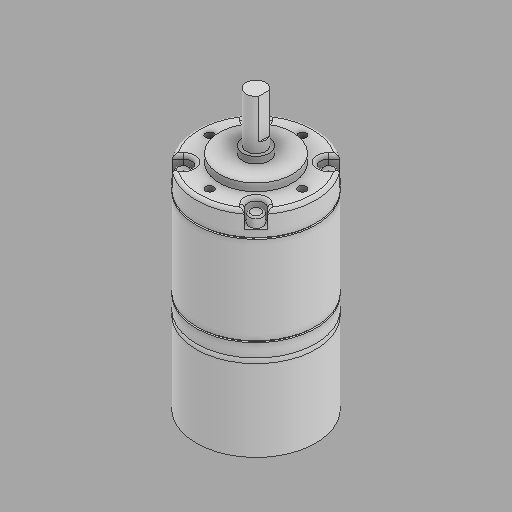
# Autodesk Inventor part: BLDC_3626
Saved by Autodesk Inventor 2025 (Build 290162000, 162)
## iProperties
Created: 2025-04-08
Part Number: BLDC_3626
Material: Типовые
Document SubType Name: Modeling
Designer: Artem Sannikov
Density: 1 g/cm^3
Appearance: По умолчанию
Author: Artem Sannikov
Autodesk Inventor part; units mm, degrees
ref_plane "YZ Plane" through (0, 0, 0) normal (1, 0, 0) x (0, 1, 0)
ref_plane "XZ Plane" through (0, 0, 0) normal (0, 1, 0) x (-1, 0, 0)
ref_plane "XY Plane" through (0, 0, 0) normal (0, 0, 1) x (1, 0, 0)
sketch "Эскиз1" plane through (0, 0, 0) normal (1, 0, 0) x (0, 1, 0)
  line L0 (0, 0) -> (734.8739, 0) construction
  line L1 (0, 0) -> (26, 0)
  line L2 (26, 0) -> (26, -16.5)
  line L3 (24.5, -18) -> (0, -18)
  line L4 (0, -18) -> (0, -6.5)
  arc A0 (24.5, -18) -> (26, -16.5) centre (24.5, -16.5) ccw
  line L5 (0, 0) -> (-3, 0)
  line L6 (-3, 0) -> (-3, -6.5)
  line L7 (-3, -6.5) -> (0, -6.5)
  line L8 (6.8488, -18) -> (80.5984, -18) construction
  line L9 (26, 0) -> (64.5, 0)
  line L10 (64.5, -11) -> (64.5, -18)
  line L11 (26, -18) -> (26, 0)
  line L12 (30.5, -18) -> (30.5, -17.5)
  line L13 (30.5, -17.5) -> (30, -17.5)
  line L14 (30, -17.5) -> (30, -18)
  line L15 (57, -18) -> (57, -17.5)
  line L16 (57, -17.5) -> (57.5, -17.5)
  line L17 (57.5, -17.5) -> (57.5, -18)
  line L18 (64.5, 0) -> (66.8, 0)
  line L19 (66.8, 0) -> (66.8, -11)
  line L20 (66.8, -11) -> (64.5, -11)
  line L21 (64.5, -18) -> (57.5, -18)
  line L22 (57, -18) -> (30.5, -18)
  line L23 (30, -18) -> (26, -18)
  line L24 (66.8, 0) -> (83.8, 0)
  line L25 (83.8, 0) -> (83.8, -3)
  line L26 (83.8, -3) -> (68.8, -3)
  line L27 (66.8, -3) -> (66.8, 0)
  line L28 (66.8, 0) -> (68.8, 0)
  line L29 (68.8, -3) -> (68.8, -4)
  line L30 (68.8, -4) -> (66.8, -4)
  line L31 (66.8, -4) -> (66.8, 0)
  line L32 (-3, -1.55) -> (-3.9167, -1.55)
  line L33 (-3.9167, -1.55) -> (-3.9167, 0)
  line L34 (-3.9167, 0) -> (-3, 0)
  point P0 (26, -18)
  point P1 (30, -17.75)
  point P2 (30.5, -17.75)
  dimension "d0" = 26
  dimension "d1" = 18
  dimension "d2" = 1.5
  dimension "d4" = 6.5
  dimension "d5" = 3
  dimension "d6" = 38.5
  dimension "d7" = 4
  dimension "d8" = 0.5
  dimension "d14" = 11
  dimension "d15" = 2.3
  dimension "d16" = 0.5
  dimension "d17" = 0.5
  dimension "d18" = 7
  dimension "d19" = 0.5
  dimension "d20" = 17
  dimension "d21" = 3
  dimension "d22" = 2
  dimension "d23" = 4
  dimension "d28" = 1.55
  constraints: 70 end point, 14 parallel, 8 horizontal, 8 perpendicular, 6 point on line, 2 midpoint, 2 point on circle, 2 tangent, 1 centre point
  measures "d0" distance of point (26, -18) L3.end
  measures "d1" distance of L1.end point (26, -18)
  measures "d2" radius of A0
  measures "d4" distance of L5.end L6.end
  measures "d5" distance between parallel lines of L4 L6
  measures "d6" distance of L10.end L11.start
  measures "d7" distance from line of point (30, -17.75) L11
  measures "d8" distance of point (30.5, -17.75) point (30, -17.75)
  measures "d14" distance of L18.end L19.end
  measures "d15" distance between parallel lines of L19 L10
  measures "d16" distance of L15.end L16.end
  measures "d17" distance of L16.end L17.end
  measures "d18" distance between parallel lines of L10 L17
  measures "d19" distance between parallel lines of L8 L13
  measures "d20" distance of L25.end L27.start
  measures "d21" distance between parallel lines of L0 L26
  measures "d22" distance of L29.end L30.end
  measures "d23" distance of L28.end L29.end
  measures "d28" distance between parallel lines of L32 L34
revolve "Вращение1" add sketch "Эскиз1" angle 360 about axis through (0, 0, 0) along (0, 1, 0)
sketch "Эскиз2" plane through (0, 83.8, 0) normal (0, 1, 0) x (1, 0, 0)
  circle A0 centre (0, 0) radius 3 projected
  line L0 (2.5, -1.6583) -> (5.0866, -1.6583)
  line L1 (5.0866, -1.6583) -> (5.0866, 2.9667)
  line L2 (5.0866, 2.9667) -> (2.5, 2.9667)
  line L3 (2.5, 2.9667) -> (2.5, -1.6583)
  point P0 (2.5, 1.6583)
  dimension "d25" = 5.5
  constraints: 8 end point, 2 parallel, 1 horizontal, 1 perpendicular, 2 other
extrude "Выдавливание1" cut sketch "Эскиз2" against normal blind 12 contours L3 A0 picked at (2.5914, 0.3806)
sketch "Эскиз3" plane through (0, 64.5, 0) normal (0, 1, 0) x (1, 0, 0)
  circle A0 centre (0, 0) radius 14 construction
  point P0 (0, 14)
  point P1 (-14, 0)
  point P2 (0, -14)
  point P3 (14, 0)
  dimension "d29" = 28
  dimension "d32" = 360
  constraints: 1 coincident, 1 vertical alignment, 7 other
hole "Отверстие1" at (0, 64.5, -14) at (-14, 64.5, 0) at (0, 64.5, 14) at (14, 64.5, 0) direction (0, -1, 0) diameter 2.459 depth 8.8 tip angle 118 thread size "M3x0.5" class "6H" standard "ISO Metric profile"
sketch "Эскиз4" plane through (0, 64.5, 0) normal (0, 1, 0) x (1, 0, 0)
  line L0 (0, 0) -> (18, 0) construction
  circle A0 centre (0, 0) radius 18 projected
  line L1 (0, 0) -> (12.7279, 12.7279) construction
  circle A1 centre (10.9602, 10.9602) radius 2.5
  line L2 (12.7279, 9.1924) -> (14.3723, 10.8368)
  line L3 (9.1924, 12.7279) -> (10.8368, 14.3723)
  line L4 (10.8368, 14.3723) -> (14.3723, 14.3723)
  line L5 (14.3723, 14.3723) -> (14.3723, 10.8368)
  line L6 (14.3723, 10.8368) -> (10.8368, 10.8368)
  line L7 (10.8368, 10.8368) -> (10.8368, 14.3723)
  line L8 (-9.1924, 12.7279) -> (-10.8368, 14.3723)
  circle A2 centre (-10.9602, 10.9602) radius 2.5
  line L9 (-10.8368, 14.3723) -> (-10.8368, 10.8368)
  line L10 (-10.8368, 10.8368) -> (-14.3723, 10.8368)
  line L11 (-12.7279, 9.1924) -> (-14.3723, 10.8368)
  line L12 (-14.3723, 10.8368) -> (-14.3723, 14.3723)
  line L13 (-14.3723, 14.3723) -> (-10.8368, 14.3723)
  line L14 (-12.7279, -9.1924) -> (-14.3723, -10.8368)
  circle A3 centre (-10.9602, -10.9602) radius 2.5
  line L15 (-14.3723, -10.8368) -> (-10.8368, -10.8368)
  line L16 (-10.8368, -10.8368) -> (-10.8368, -14.3723)
  line L17 (-9.1924, -12.7279) -> (-10.8368, -14.3723)
  line L18 (-10.8368, -14.3723) -> (-14.3723, -14.3723)
  line L19 (-14.3723, -14.3723) -> (-14.3723, -10.8368)
  line L20 (9.1924, -12.7279) -> (10.8368, -14.3723)
  circle A4 centre (10.9602, -10.9602) radius 2.5
  line L21 (10.8368, -14.3723) -> (10.8368, -10.8368)
  line L22 (10.8368, -10.8368) -> (14.3723, -10.8368)
  line L23 (12.7279, -9.1924) -> (14.3723, -10.8368)
  line L24 (14.3723, -10.8368) -> (14.3723, -14.3723)
  line L25 (14.3723, -14.3723) -> (10.8368, -14.3723)
  point P0 (-12.7279, 12.7279)
  point P1 (-12.7279, -12.7279)
  point P2 (12.7279, -12.7279)
  dimension "d41" = 45
  dimension "d42" = 5
  dimension "d45" = 360
  constraints: 52 end point, 16 point on circle, 4 centre point, 4 parallel, 2 horizontal, 1 perpendicular, 1 point on line, 61 other
  measures "d41" angle of L1 L0
  measures "d42" diameter of A1
extrude "Выдавливание2" cut sketch "Эскиз4" against normal blind 5 contours L6 A1 A0 | L2 A1 L6 | A0 A4 L22 | L22 A4 L23 | A1 L7 A0 | A1 L6 L7 | A1 L7 L6 | A0 L21 A4 | A4 L21 L22 | L22 L21 A4 | L7 A1 L3 | L20 A4 L21 | L9 A2 A0 | L8 A2 L9 | A0 A3 L16 | L16 A3 L17 | A2 L10 A0 | A2 L9 L10 | A2 L10 L9 | A0 L15 A3 | A3 L15 L16 | L16 L15 A3 | L10 A2 L11 | L14 A3 L15
fillet "Сопряжение1" radius 1 17 edges at (5.7139, 64.5, -17.069) (-5.7139, 64.5, -17.069) (-18, 64.5, 0) (0, 64.5, 18) (18, 64.5, 0) (10.0146, 64.5, -13.5501) (13.5501, 64.5, -10.0146) (9.1924, 64.5, -9.1924) (13.5501, 64.5, 10.0146) (10.0146, 64.5, 13.5501) (9.1924, 64.5, 9.1924) (-13.5501, 64.5, -10.0146) (-10.0146, 64.5, -13.5501) (-9.1924, 64.5, -9.1924) (-10.0146, 64.5, 13.5501) (-13.5501, 64.5, 10.0146) (-9.1924, 64.5, 9.1924)
sketch "Эскиз5" plane through (0, 59.5, 0) normal (0, 1, 0) x (1, 0, 0)
  arc A0 (-12.7279, 9.1924) -> (-9.1924, 12.7279) centre (-10.9602, 10.9602) ccw construction
  circle A1 centre (-10.9602, 10.9602) radius 2
  circle A2 centre (-10.9602, -10.9602) radius 2
  circle A3 centre (10.9602, -10.9602) radius 2
  circle A4 centre (10.9602, 10.9602) radius 2
  point P0 (0, 0)
  dimension "d50" = 4
  dimension "d53" = 360
  constraints: 4 centre point, 1 coincident, 9 other
  measures "d50" diameter of A1
extrude "Выдавливание3" add sketch "Эскиз5" along normal blind 3
fillet "Сопряжение2" radius 0.5 4 edges at (8.9602, 62.5, -10.9602) (-12.9602, 62.5, -10.9602) (-12.9602, 62.5, 10.9602) (8.9602, 62.5, 10.9602)
